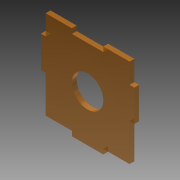
# Autodesk Inventor part: SideB
Saved by Autodesk Inventor 2014 (Build 180170000, 170)
## iProperties
Created: 2014-11-21
Part Number: SideB
Material: Generic
Document SubType Name: Modeling
Designer: JLM
Density: 1 g/cm^3
Appearance: Default
Author: JLM
Autodesk Inventor part; units mm, degrees
ref_plane "YZ Plane" through (0, 0, 0) normal (1, 0, 0) x (0, 1, 0)
ref_plane "XZ Plane" through (0, 0, 0) normal (0, 1, 0) x (-1, 0, 0)
ref_plane "XY Plane" through (0, 0, 0) normal (0, 0, 1) x (1, 0, 0)
sketch "Sketch1" plane through (0, 0, 0) normal (0, 0, 1) x (1, 0, 0)
  line L0 (-28.321, -28.321) -> (28.321, -28.321)
  line L1 (28.321, -28.321) -> (28.321, 28.321)
  line L2 (28.321, 28.321) -> (-28.321, 28.321)
  line L3 (-28.321, 28.321) -> (-28.321, -28.321)
  line L4 (-28.321, -28.321) -> (28.321, 28.321) construction
  line L5 (28.321, -28.321) -> (-28.321, 28.321) construction
  point P0 (0, 0)
  dimension "d0" = 56.642
  dimension "d1" = 56.642
  constraints: 12 end point, 2 midpoint, 2 parallel, 1 horizontal, 1 perpendicular
  measures "d0" distance of L2.end L1.end
  measures "d1" distance of L1.end L0.end
extrude "Extrusion1" add sketch "Sketch1" against normal blind 2.921
sketch "Sketch4" plane through (0, 0, 0) normal (0, 0, 1) x (1, 0, 0)
  line L0 (-28.321, -28.321) -> (-9.525, -28.321)
  line L1 (-9.525, -28.321) -> (-9.525, -25.4)
  line L2 (-9.525, -25.4) -> (-28.321, -25.4)
  line L3 (-28.321, -25.4) -> (-28.321, -28.321)
  line L4 (28.321, 28.321) -> (-28.321, 28.321) projected
  line L5 (-28.321, 28.321) -> (-28.321, -28.321) projected
  line L6 (-9.525, 28.321) -> (9.525, 28.321)
  line L7 (9.525, 28.321) -> (9.525, 25.4)
  line L8 (9.525, 25.4) -> (-9.525, 25.4)
  line L9 (-9.525, 25.4) -> (-9.525, 28.321)
  line L10 (-28.321, -28.321) -> (-25.4, -28.321)
  line L11 (-25.4, -28.321) -> (-25.4, -2.921)
  line L12 (-25.4, -2.921) -> (-28.321, -2.921)
  line L13 (-28.321, -2.921) -> (-28.321, -28.321)
  line L14 (-28.321, 28.321) -> (-25.4, 28.321)
  line L15 (-25.4, 28.321) -> (-25.4, 16.129)
  line L16 (-25.4, 16.129) -> (-28.321, 16.129)
  line L17 (-28.321, 16.129) -> (-28.321, 28.321)
  line L18 (0, -3.175) -> (0, -6.3407)
  line L19 (28.321, -28.321) -> (9.525, -28.321)
  line L20 (9.525, -28.321) -> (9.525, -25.4)
  line L21 (9.525, -25.4) -> (28.321, -25.4)
  line L22 (28.321, -25.4) -> (28.321, -28.321)
  line L23 (28.321, 28.321) -> (28.321, -28.321)
  line L24 (9.525, 25.4) -> (9.525, 28.321)
  line L25 (28.321, -28.321) -> (25.4, -28.321)
  line L26 (25.4, -28.321) -> (25.4, -2.921)
  line L27 (25.4, -2.921) -> (28.321, -2.921)
  line L28 (28.321, -2.921) -> (28.321, -28.321)
  line L29 (28.321, 28.321) -> (25.4, 28.321)
  line L30 (25.4, 28.321) -> (25.4, 16.129)
  line L31 (25.4, 16.129) -> (28.321, 16.129)
  line L32 (28.321, 16.129) -> (28.321, 28.321)
  line L33 (-28.321, -28.321) -> (28.321, -28.321) projected
  point P0 (0, 0)
  point P1 (28.321, 0.1976)
  dimension "d16" = 2.921
  dimension "d37" = 9.525
  dimension "d38" = 18.796
  dimension "d44" = 2.921
  dimension "d45" = 19.05
  dimension "d46" = 18.796
  dimension "d53" = 25.4
  dimension "d54" = 19.05
  dimension "d55" = 2.921
  dimension "d56" = 2.921
  dimension "d57" = 12.192
  dimension "d58" = 18.796
  dimension "d59" = 19.05
  dimension "d60" = 12.192
  dimension "d61" = 19.05
  dimension "d62" = 25.4
  constraints: 62 end point, 11 symmetric about line, 9 parallel, 4 horizontal, 4 perpendicular, 2 point on line, 1 collinear
  measures "d16" distance of L0.end L1.end
  measures "d37" distance from line of point (0, 0) L1
  measures "d38" distance of L0.start L0.end
  measures "d44" distance of L8.end L6.start
  measures "d45" distance of L7.end L8.end
  measures "d46" distance between parallel lines of L5 L9
  measures "d53" distance of L11.end L10.end
  measures "d54" distance between parallel lines of L12 L16
  measures "d55" distance of L15.end L16.end
  measures "d56" distance of L11.end L12.end
  measures "d57" distance of L14.end L15.end
  measures "d58" distance between parallel lines of L28 L20
  measures "d59" distance between parallel lines of L20 L1
  measures "d60" distance between parallel lines of L31 L4
  measures "d61" distance between parallel lines of L27 L31
  measures "d62" distance between parallel lines of L33 L27
extrude "Extrusion5" cut sketch "Sketch4" against normal blind 25.4 contours L3 L2 L11 L0 | L11 L2 L1 L0 | L5 L12 L11 L2 | L20 L21 L26 L19 | L5 L4 L15 L16 | L26 L21 L22 L19 | L26 L27 L23 L21 | L4 L7 L8 L9 | L31 L30 L4 L23
hole "Hole1" at (0, 0, 0) direction (0, 0, -1) diameter 19.05 end through all
equation "\"d1\" = d0"
equation "\"d38\" = -d37 + 0.5 * d0"
equation "\"d44\" = d16"
equation "\"d45\" = d42"
equation "\"d46\" = d38"
equation "\"d55\" = d16"
equation "\"d56\" = d16"
equation "\"d59\" = d45"
equation "\"d19\" = 0.5 * d0"
equation "\"d48\" = 0.5 * d0"
equation "\"d42\" = 2 * d37"
body "Solid1"
